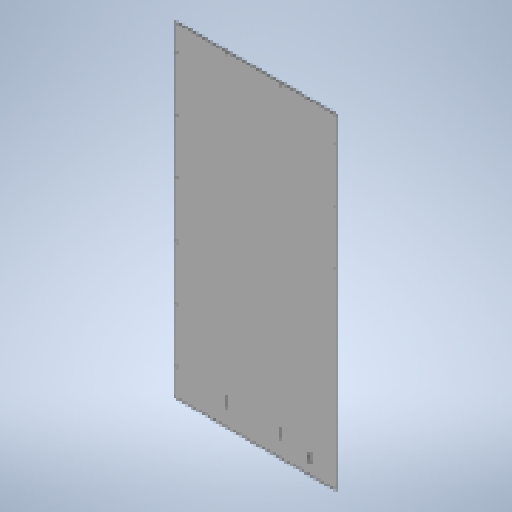
# Autodesk Inventor part: GBK 1325 shield 1.2
Saved by Autodesk Inventor 2026 (Build 300175000, 175)
## iProperties
Created: 2026-04-17
Part Number: GBK 1325 shield 1.2
Material: Steel
Document SubType Name: Sheet Metal
Designer: admin
Stock Number: 1329
Mass: 138487 g
Surface Area: 88564.8 cm^2
Volume: 17641.6 cm^3
Density: 7.85 g/cm^3
Flat Pattern Width: 148 cm
Flat Pattern Length: 298 cm
Flat Pattern Area: 44104 cm^2
Sheet Metal Rule: По умолчанию_мм
Sheet Metal Width: 1480,000 мм
Sheet Metal Length: 2980,000 мм
Sheet Metal Area: 4410400,000 мм^2
Appearance: Default
Author: admin
Autodesk Inventor part; units mm, degrees
ref_plane "YZ Plane" through (0, 0, 0) normal (1, 0, 0) x (0, 1, 0)
ref_plane "XZ Plane" through (0, 0, 0) normal (0, 1, 0) x (-1, 0, 0)
ref_plane "XY Plane" through (0, 0, 0) normal (0, 0, 1) x (1, 0, 0)
sketch "Sketch1" plane through (0, 0, 0) normal (0, 0, 1) x (1, 0, 0)
  line L0 (740, -1490) -> (-740, -1490)
  line L1 (-740, -1490) -> (-740, 1490)
  line L2 (-740, 1490) -> (740, 1490)
  line L3 (740, 1490) -> (740, -1490)
  line L4 (740, -1490) -> (-740, 1490) construction
  line L5 (-740, -1490) -> (740, 1490) construction
  point P0 (0, 0)
  dimension "d0" = 1480
  dimension "d1" = 2980
  measures "d0" distance of L1.end L2.end
  measures "d1" distance of L0.end L1.end
extrude "Plate2" add sketch "Sketch1" along normal blind 4
sketch "Sketch4" plane through (0, 0, 4) normal (0, 0, 1) x (1, 0, 0)
  line L0 (507.8568, -1305.8232) -> (507.8568, -1663.5137) construction
  line L1 (507.8568, -1663.5137) -> (476.5926, -1663.5137) construction
  line L2 (476.5926, -1663.5137) -> (476.5926, -1305.8232) construction
  line L3 (476.5926, -1305.8232) -> (507.8568, -1305.8232) construction
  line L4 (710, -1236.5) -> (710, -1232.5) projected
  line L5 (710, -739.8333) -> (710, -735.8333) projected
  line L6 (710, -243.1667) -> (710, -239.1667) projected
  line L7 (710, 253.5) -> (710, 257.5) projected
  line L8 (710, 750.1667) -> (710, 754.1667) projected
  line L9 (710, 1246.8333) -> (710, 1250.8333) projected
  line L10 (230.5109, -1240) -> (230.5109, -1337) projected
  line L11 (230.5109, -1337) -> (226.5119, -1337) projected
  line L12 (-269.6177, -1240) -> (-269.6177, -1337) projected
  line L13 (-269.6177, -1337) -> (-273.6167, -1337) projected
  line L14 (-739.3197, -1236.5) -> (-710, -1236.5) projected
  line L15 (-710, -1236.5) -> (-710, -1232.5) projected
  line L16 (-739.3197, -739.8333) -> (-710, -739.8333) projected
  line L17 (-710, -739.8333) -> (-710, -735.8333) projected
  line L18 (-739.3197, -243.1667) -> (-710, -243.1667) projected
  line L19 (-710, -243.1667) -> (-710, -239.1667) projected
  line L20 (-739.3197, 253.5) -> (-710, 253.5) projected
  line L21 (-710, 253.5) -> (-710, 257.5) projected
  line L22 (-739.3197, 750.1667) -> (-710, 750.1667) projected
  line L23 (-710, 750.1667) -> (-710, 754.1667) projected
  line L24 (-739.3197, 1246.8333) -> (-710, 1246.8333) projected
  line L25 (-710, 1246.8333) -> (-710, 1250.8333) projected
  ellipse E0 centre (-269.6177, 1488) end of major axis (-269.6177, 1518) minor radius 0.6803 (-269.6177, 1458) -> (-269.6177, 1518) ccw projected
  line L26 (-269.6177, 1458) -> (-273.6167, 1458) projected
  ellipse E1 centre (230.5109, 1488) end of major axis (230.5109, 1518) minor radius 0.6803 (230.5109, 1458) -> (230.5109, 1518) ccw projected
  line L27 (230.5109, 1458) -> (226.5119, 1458) projected
  point P0 (0, 0)
  constraints: 4 other
mark "Mark2"
equation "\"d0\" = Лист_ширина"
equation "\"d3\" = Thickness"
equation "\"BendRadius\" = Thickness"
equation "\"BendReliefWidth\" = Thickness"
equation "\"BendReliefDepth\" = 0.5 * Thickness"
equation "\"CornerReliefSize\" = 4 * Thickness"
equation "\"MinimumRemnant\" = 2 * Thickness"
equation "\"TransitionRadius\" = BendRadius"
equation "\"JacobiRadiusSize\" = BendRadius"
equation "\"GapSize\" = Thickness"
equation "\"Лист_ширина\" = 1480"
equation "\"Thickness\" = 4"
body "Solid2"
